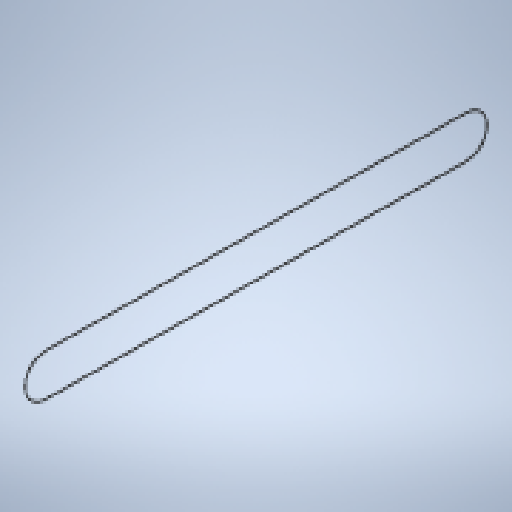
# Autodesk Inventor part: Elastic
Saved by Autodesk Inventor 2023 (Build 270158000, 158)
## iProperties
Created: 2022-11-07
Part Number: Elastic
Material: Acetal Resin, Black
Document SubType Name: Modeling
Designer: D.C. Eksteen
Density: 1.425 g/cm^3
Appearance: Smooth - Black
Author: D.C. Eksteen
Autodesk Inventor part; units mm, degrees
ref_plane "YZ Plane" through (0, 0, 0) normal (1, 0, 0) x (0, 1, 0)
ref_plane "XZ Plane" through (0, 0, 0) normal (0, 1, 0) x (-1, 0, 0)
ref_plane "XY Plane" through (0, 0, 0) normal (0, 0, 1) x (1, 0, 0)
sketch "Sketch1" plane through (0, 0, 0) normal (1, 0, 0) x (0, 1, 0)
  circle A0 centre (-87.2391, 327.4627) radius 48 projected
  circle A1 centre (-97.2391, -669.9464) radius 48 projected
  line L0 (-39.2415, 326.9815) -> (-49.2415, -670.4276)
  line L1 (-145.2367, -669.4652) -> (-135.2367, 327.9439)
  arc A2 (-145.2367, -669.4652) -> (-49.2415, -670.4276) centre (-97.2391, -669.9464) ccw
  arc A3 (-39.2415, 326.9815) -> (-135.2367, 327.9439) centre (-87.2391, 327.4627) ccw
  line L2 (-45.2417, -670.4677) -> (-35.2417, 326.9414)
  arc A4 (-35.2417, 326.9414) -> (-139.2365, 327.984) centre (-87.2391, 327.4627) ccw
  line L3 (-139.2365, 327.984) -> (-149.2365, -669.4251)
  arc A5 (-149.2365, -669.4251) -> (-45.2417, -670.4677) centre (-97.2391, -669.9464) ccw
  point P0 (0, 0)
  dimension "d0" = 4
  constraints: 12 point on circle, 8 end point, 8 tangent, 4 centre point, 3 other
  measures "d0" distance between parallel lines of L0 L2
extrude "Extrusion1" add sketch "Sketch1" along normal blind 4
fillet "Fillet1" radius 2 12 edges at (4, -40.2417, -171.7632) (4, -86.7178, 379.4601) (4, -144.2365, -170.7205) (4, -97.7604, -721.9438) (0, -86.7178, 379.4601) (0, -144.2365, -170.7205) (0, -97.7604, -721.9438) (0, -40.2417, -171.7632) (0, -97.7203, -717.944) (0, -140.2367, -170.7606) (0, -86.7579, 375.4603) (0, -44.2415, -171.7231)
fillet "Fillet2" radius 1.7 4 edges at (4, -86.7579, 375.4603) (4, -44.2415, -171.7231) (4, -97.7203, -717.944) (4, -140.2367, -170.7606)
body "Solid1"
